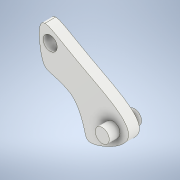
# Autodesk Inventor part: Component20
Saved by Autodesk Inventor 2022 (Build 260153000, 153)
## iProperties
Created: 2022-01-29
Part Number: Component20
Material: Generic
Document SubType Name: Modeling
Designer: Administrator
Density: 1 g/cm^3
Appearance: Default
Title: Component20
Author: Administrator
Autodesk Inventor part; units mm, degrees
ref_plane "YZ Plane" through (0, 0, 0) normal (1, 0, 0) x (0, 1, 0)
ref_plane "XZ Plane" through (0, 0, 0) normal (0, 1, 0) x (-1, 0, 0)
ref_plane "XY Plane" through (0, 0, 0) normal (0, 0, 1) x (1, 0, 0)
sketch "Sketch2" plane through (0, 0, 0) normal (0, 0, 1) x (1, 0, 0)
  circle A0 centre (16.3843, -7.9628) radius 3.25
  circle A1 centre (-12.7448, 12.0118) radius 3.25
  spline S0 degree 5 poles (-15.1962, 18.7561) (-14.5896, 18.7561) (-13.2026, 18.4351) (-10.6346, 17.1323) (-6.4651, 14.6996) (-0.2822, 11.1656) (6.4599, 7.6357) (13.2891, 4.0668) (19.3766, 0.3) (23.7562, -3.8471) (24.4838, -8.3749) (20.3318, -12.8685) (13.6646, -16.602) (7.3971, -18.7975) (4.0638, -18.8679) (3.624, -16.5838) (2.5621, -12.4761) (0.7686, -8.0745) (-1.4681, -4.703) (-3.5615, -3.0667) (-6.896, -1.5503) (-10.8175, -0.2618) (-14.0493, 0.5077) (-15.7407, 1.3524) (-17.1518, 5.8178) (-18.0494, 12.3374) (-17.8489, 16.8489) (-16.8428, 18.4351) (-15.8029, 18.7561) (-15.1962, 18.7561) knots 0 0 0 0 0 0 0.04 0.08 0.12 0.16 0.2 0.24 0.28 0.32 0.36 0.4 0.44 0.48 0.52 0.56 0.6 0.64 0.68 0.72 0.76 0.8 0.84 0.88 0.92 0.96 1 1 1 1 1 1 weights 1 1 1 1 1 1 1 1 1 1 1 1 1 1 1 1 1 1 1 1 1 1 1 1 1 1 1 1 1 1
  point P0 (0, 0)
  dimension "d6" = 6.5
  constraints: 2 centre point, 1 equal radius, 1 other
  measures "d6" diameter of A1
extrude "Extrusion1" add sketch "Sketch2" along normal blind 5 contours A0 | S0
extrude "Extrusion2" add sketch "Sketch2" against normal blind 5 contours A0
sketch "Sketch3" plane through (0, 0, 5) normal (0, 0, 1) x (1, 0, 0)
  circle A0 centre (16.3843, -7.9628) radius 3.25 projected
  circle A1 centre (-12.7448, 12.0118) radius 3.25 projected
  point P0 (0, 0)
  constraints: 1 other
extrude "Extrusion3" add sketch "Sketch3" along normal blind 5 contours A0
equation "\"d6\" = R"
equation "\"d0\" = thickness"
equation "\"d2\" = thickness"
equation "\"d4\" = thickness"
equation "\"R\" = 6.5"
equation "\"thickness\" = 5"
equation "\"width\" = 6.5"
equation "\"R1\" = 9"
body "Solid1"
